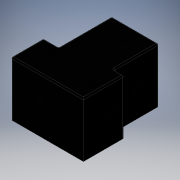
# Autodesk Inventor part: JTN1AS-PA-F-DC5V_Relay
Saved by Autodesk Inventor 2016 (Build 200138000, 138)
## iProperties
Created: 2016-09-07
Part Number: JTN1AS-PA-F-DC5V_Relay
Material: Generic
Document SubType Name: Modeling
Designer: jfixelle
Density: 1 g/cm^3
Appearance: Black
Author: jfixelle
Autodesk Inventor part; units mm, degrees
ref_plane "YZ Plane" through (0, 0, 0) normal (1, 0, 0) x (0, 1, 0)
ref_plane "XZ Plane" through (0, 0, 0) normal (0, 1, 0) x (-1, 0, 0)
ref_plane "XY Plane" through (0, 0, 0) normal (0, 0, 1) x (1, 0, 0)
sketch "Sketch1" plane through (0, 0, 0) normal (0, 1, 0) x (-1, 0, 0)
  line L0 (13.75, 16.25) -> (-13.75, 16.25)
  line L1 (-13.75, 16.25) -> (-13.75, -16.25)
  line L2 (-13.75, -16.25) -> (13.75, -16.25)
  line L3 (13.75, -16.25) -> (13.75, 16.25)
  line L4 (-13.75, 0.7762) -> (-9.8958, 0.7762)
  line L5 (-9.8958, 0.7762) -> (-9.8958, -16.25)
  line L6 (13.75, 3.9572) -> (7.9724, 3.9572)
  line L7 (7.9724, 3.9572) -> (7.9724, -16.25)
  point P0 (0, 0)
  dimension "d0" = 27.5
  dimension "d1" = 13.75
  dimension "d2" = 32.5
  dimension "d3" = 16.25
  constraints: 16 end point, 4 point on line, 3 horizontal, 3 perpendicular, 2 parallel
  measures "d0" distance of L0.start L0.end
  measures "d1" distance from line of point (0, 0) L3
  measures "d2" distance of L2.end L0.start
  measures "d3" distance from line of point (0, 0) L2
extrude "Extrusion1" add sketch "Sketch1" along normal blind 20.8 contours L3 L6 L7 L2 L5 L4 L1 L0
sketch "Sketch2" plane through (0, 0, 0) normal (0, -1, 0) x (1, 0, 0)
  circle A0 centre (-8.89, 7.62) radius 0.8
  circle A1 centre (8.89, 5.08) radius 0.8
  circle A2 centre (-5.08, -7.62) radius 0.32
  circle A3 centre (5.08, -7.62) radius 0.32
  point P0 (0, 0)
  dimension "d6" = 0.64
  dimension "d7" = 0.64
  dimension "d8" = 3.81
  dimension "d9" = 13.97
  dimension "d10" = 17.78
  dimension "d11" = 2.54
  dimension "d12" = 15.24
  dimension "d13" = 0
  dimension "d14" = 5.08
  dimension "d15" = 7.62
  dimension "d16" = 1.6
  dimension "d17" = 1.6
  constraints: 4 centre point
  measures "d6" diameter of A3
  measures "d7" diameter of A2
  measures "d8" horizontal distance of A2.centre A0.centre
  measures "d9" horizontal distance of A3.centre A0.centre
  measures "d10" horizontal distance of A1.centre A0.centre
  measures "d11" vertical distance of A1.centre A0.centre
  measures "d12" vertical distance of A2.centre A0.centre
  measures "d13" vertical distance of A2.centre A3.centre
  measures "d14" horizontal distance of point (0, 0) A2.centre
  measures "d15" vertical distance of point (0, 0) A2.centre
  measures "d16" diameter of A0
  measures "d17" diameter of A1
extrude "Extrusion2" add sketch "Sketch2" along normal blind 3.6
fillet "Fillet1" radius 0.5 15 edges at (-7.9724, 10.4, 3.9572) (-7.9724, 10.4, -16.25) (-13.75, 10.4, 3.9572) (-13.75, 10.4, 16.25) (9.8958, 10.4, -16.25) (13.75, 10.4, 0.7762) (9.8958, 10.4, 0.7762) (0, 20.8, 16.25) (-13.75, 20.8, 10.1036) (-10.8612, 20.8, 3.9572) (-7.9724, 20.8, -6.1464) (0.9617, 20.8, -16.25) (9.8958, 20.8, -7.7369) (11.8229, 20.8, 0.7762) (13.75, 20.8, 8.5131)
body "Solid1"
